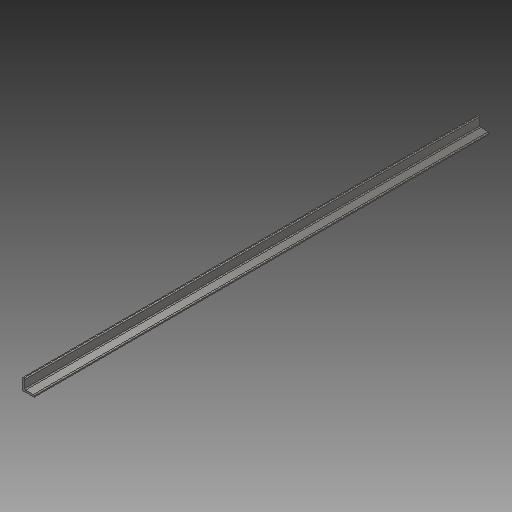
# Autodesk Inventor part: 60in1.5Lch
Saved by Autodesk Inventor 2018 (Build 220112000, 112)
## iProperties
Created: 2018-07-30
Part Number: 60in1.5Lch
Material: Steel, Mild
Document SubType Name: Modeling
Designer: Cole Tucker
Density: 7.85 g/cm^3
Appearance: Semi-Polished
Mass: 5280.46 g
Surface Area: 2269.1 cm^2
Volume: 672.669 cm^3
Author: Cole Tucker
Autodesk Inventor part; units mm, degrees
ref_plane "YZ Plane" through (0, 0, 0) normal (1, 0, 0) x (0, 1, 0)
ref_plane "XZ Plane" through (0, 0, 0) normal (0, 1, 0) x (-1, 0, 0)
ref_plane "XY Plane" through (0, 0, 0) normal (0, 0, 1) x (1, 0, 0)
sketch "Sketch1" plane through (0, 0, 0) normal (0, 0, 1) x (1, 0, 0)
  line L0 (0, 0) -> (38.1, 0)
  line L1 (38.1, 0) -> (38.1, 38.1)
  line L2 (38.1, 38.1) -> (0, 38.1)
  line L3 (0, 38.1) -> (0, 0)
  line L4 (0, 38.1) -> (6.35, 38.1)
  line L5 (38.1, 0) -> (38.1, 6.35)
  line L6 (0, 0) -> (6.35, 0)
  line L7 (6.35, 0) -> (6.35, 6.35)
  line L8 (6.35, 6.35) -> (0, 6.35)
  line L9 (0, 6.35) -> (0, 0)
  line L10 (6.35, 38.1) -> (6.35, 6.35)
  line L11 (6.35, 6.35) -> (38.1, 6.35)
  dimension "d0" = 38.1
  dimension "d1" = 38.1
  dimension "d2" = 6.35
  dimension "d3" = 6.35
  dimension "d4" = 6.35
  dimension "d5" = 6.35
  constraints: 24 end point, 4 parallel, 2 horizontal, 2 perpendicular, 2 point on line
  measures "d0" distance of L2.end L1.end
  measures "d1" distance of L1.end L0.end
  measures "d2" distance of L2.end L4.end
  measures "d3" distance of L0.end L5.end
  measures "d4" distance of L8.end L7.end
  measures "d5" distance of L7.end L6.end
extrude "Extrusion1" add sketch "Sketch1" along normal blind 1524 contours L3 L8 L7 L0 | L7 L11 L1 L0 | L3 L2 L10 L8
fillet "Fillet1" radius 3.175 3 edges at (6.35, 38.1, 762) (38.1, 6.35, 762) (6.35, 6.35, 762)
body "Solid1"
